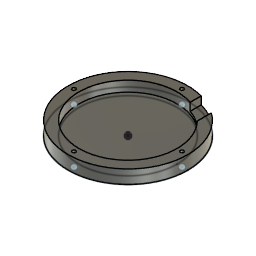
Hackpad (Autodesk Fusion 360 design; units mm, degrees)
Autodesk Fusion 360 part; units mm, degrees
sketch "Sketch1" plane through (0, 0, 0) normal (0, 0, 1) x (1, 0, 0)
  circle A0 centre (0, 0) radius 47.225
  circle A1 centre (0, 0) radius 57.5
  circle A2 centre (0, 52) radius 1.7
  circle A3 centre (0, -52) radius 1.7
  circle A4 centre (-52, 0) radius 1.7
  circle A5 centre (52, 0) radius 1.7
  dimension "d1" = 94.45
  dimension "d2" = 115
  dimension "d3" = 3.4
  dimension "d4" = 3.4
  dimension "d5" = 3.4
  dimension "d6" = 3.4
  constraint coincident A0.centre A1.centre
  measures "d1" diameter of A0
  measures "d2" diameter of A1
  measures "d3" diameter of A2
  measures "d4" diameter of A3
  measures "d5" diameter of A4
  measures "d6" diameter of A5
extrude "Extrude4" add sketch "Sketch1" along normal blind 3.1 contours A2 | A3 | A4 | A5 makes body 1 at (53.6979, -0.0847, 2.0667) makes body 2 at (-50.3021, -0.0847, 2.0667) makes body 3 at (-1.5975, 52.5814, 2.0667) makes body 4 at (-1.5975, -51.4186, 2.0667)
extrude "Extrude5" add sketch "Sketch1" along normal blind 13 bodies 1 2 3 4
extrude "Extrude6" add sketch "Sketch1" along normal blind 3 contours A0 bodies 1
sketch "Sketch2" plane through (0, 0, 13) normal (0, 0, 1) x (-1, 0, 0)
  circle A0 centre (0, -52) radius 1.7
  circle A1 centre (52, 0) radius 1.7
  circle A2 centre (0, 52) radius 1.7
  circle A3 centre (-52, 0) radius 1.7
  circle A4 centre (0, 0) radius 47.225
  circle A5 centre (0, 0) radius 57.5
  line L0 (-15, -35) -> (-34, -35)
  line L1 (-34, -35) -> (-34, -57)
  line L2 (-34, -57) -> (-15, -57)
  line L3 (-15, -57) -> (-15, -35)
  line L4 (-34, -35) -> (-15, -35)
  line L5 (-15, -35) -> (-15, -31)
  line L6 (-15, -31) -> (-34, -31)
  line L7 (-34, -31) -> (-34, -35)
  constraint horizontal L0
  constraint vertical L1
  constraint horizontal L2
  constraint vertical L3
  constraint horizontal L4
  constraint vertical L5
  constraint horizontal L6
  constraint vertical L7
extrude "Extrude7" cut sketch "Sketch2" against normal blind 7.5 contours A4 L0 L4 L7 | A4 A5 L0 L1 L3 L4 bodies 1
extrude "Extrude3" [suppressed]
extrude "Extrude2" [suppressed]
